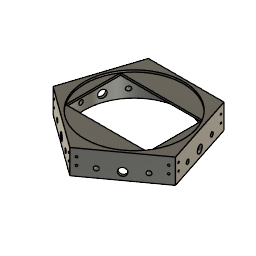
StarClock_InnerPart (Autodesk Fusion 360 design; units mm, degrees)
Autodesk Fusion 360 part; units mm, degrees
note: some values were not read from the file. Set by a fixed rule: which sketch regions a step uses.
sketch "Skizze1" plane through (0, 0, 0) normal (0, 0, 1) x (1, 0, 0)
  line L0 (0, -68.245) -> (64.9049, -21.0889)
  line L1 (64.9049, -21.0889) -> (40.1134, 55.2114)
  line L2 (40.1134, 55.2114) -> (-40.1134, 55.2114)
  line L3 (-40.1134, 55.2114) -> (-64.9049, -21.0889)
  line L4 (-64.9049, -21.0889) -> (0, -68.245)
  circle A0 centre (0, 0) radius 52.5
  line L5 (-43.5, 29) -> (43.5, 29)
  line L6 (43.5, 29) -> (43.5, -29)
  line L7 (43.5, -29) -> (-43.5, -29)
  line L8 (-43.5, -29) -> (-43.5, 29)
  line L9 (0, 0) -> (0, 29)
  line L10 (0, 29) -> (-43.5, 29)
  line L11 (0, -68.245) -> (0, -66.245)
  line L12 (0, -66.245) -> (63.0027, -20.4708)
  line L13 (63.0027, -20.4708) -> (38.9378, 53.5933)
  line L14 (38.9378, 53.5933) -> (-38.9378, 53.5933)
  line L15 (-38.9378, 53.5933) -> (-63.0027, -20.4708)
  line L16 (-63.0027, -20.4708) -> (0, -66.245)
  dimension "d1" = 68.245
  dimension "d2" = 105
  dimension "d3" = 87
  dimension "d4" = 58
  dimension "d5" = 29
  dimension "d6" = 43.5
  dimension "d7" = 2
  constraint coincident A0.centre L9.start
  constraint horizontal L5
  constraint vertical L6
  constraint horizontal L7
  constraint vertical L8
  constraint vertical L9
  constraint perpendicular L9 L10
  constraint vertical L11
  constraint coincident L11.end L12.start
  constraint coincident L9 A0.centre
  measures "d1" distance of L0.start A0.centre
  measures "d2" diameter of A0
  measures "d3" distance of L5.end L5.start
  measures "d4" distance of L7.end L5.start
  measures "d5" distance of A0.centre L9.end
  measures "d6" distance of L9.end L5.start
  measures "d7" distance of L0.start L11.end
extrude "Extrusion1" add sketch "Skizze1" along normal blind 12 and the other way blind 14 contours L0 L1 L2 L3 L4 | L12 L13 L14 L15 L16
extrude "Extrusion2" add sketch "Skizze1" along normal blind 2 from surface at 8 contours A0
sketch "Skizze2" plane through (32.4524, -44.6669, 0) normal (0.587785, -0.809017, 0) x (0.809017, 0.587785, 0)
  line L0 (40.1134, -14) -> (40.1134, 12)
  line L1 (40.1134, 12) -> (-40.1134, 12)
  line L2 (-40.1134, -14) -> (40.1134, -14)
  line L3 (0, -5) -> (-20, -5)
  circle A0 centre (-35, 4) radius 1
  line L4 (-35, -4) -> (-35, 4)
  line L5 (0, -12) -> (0, 12)
  circle A1 centre (-35, -4) radius 1
  line L6 (-35, 4) -> (-35, 12)
  line L7 (-35, -12) -> (-35, -4)
  circle A2 centre (-20, -5) radius 2.25
  line L8 (35, 4) -> (35, 12)
  circle A3 centre (35, -4) radius 1
  line L9 (35, -12) -> (35, -4)
  circle A4 centre (35, 4) radius 1
  line L10 (35, -4) -> (35, 4)
  line L11 (0, -5) -> (20, -5)
  circle A5 centre (20, -5) radius 2.25
  circle A6 centre (0, -6) radius 4
  point P0 (0, -5)
  dimension "d16" = 8
  dimension "d17" = 8
  dimension "d18" = 8
  dimension "d19" = 2
  dimension "d21" = 2
  dimension "d23" = 20
  dimension "d27" = 4.5
  constraint vertical L7
  constraint parallel L4 L7
  constraint parallel L4 L6
  constraint coincident L4.start A1.centre
  constraint coincident A0.centre L4.end
  constraint coincident P0 L3.start
  constraint perpendicular L3 L5
  constraint coincident L3.end A2.centre
  constraint symmetric L4.start L5 A3.centre
  constraint symmetric L6.end L5 L8.end
  constraint symmetric A0.centre L5 L8.start
  constraint symmetric L7.start L5 L9.start
  constraint symmetric L3.end L5 L11.end
  constraint symmetric P0 L5 L3.start
  constraint symmetric A0 L5 A4
  constraint symmetric L5 A1 A3
  constraint symmetric L5 A2 A5
  constraint coincident L5 A6.centre
  measures "d16" distance of L4.start L7.start
  measures "d17" distance of L4.start A0.centre
  measures "d18" distance of L6.end A0.centre
  measures "d19" diameter of A1
  measures "d21" diameter of A0
  measures "d23" distance of L3.end P0
  measures "d27" diameter of A2
extrude "Extrusion3" cut sketch "Skizze2" against normal blind 4 contours A0 L4 L6 | A0 L4 L6 | L4 A1 L7 | L4 A1 L7 | L8 A4 L10 | L8 A4 L10 | A3 L9 L10 | A3 L9 L10
extrude "Extrusion4" cut sketch "Skizze2" against normal blind 9 contours L3 L5 A6 | L5 L11 A6 | L3 L5 A6 | L5 L11 A6 | A2 | A5
sketch "Skizze3" plane through (32.4524, -44.6669, 0) normal (0.587785, -0.809017, 0) x (0.809017, 0.587785, 0)
sketch "Skizze4" plane through (52.5091, 17.0612, 0) normal (0.951057, 0.309017, 0) x (-0.309017, 0.951057, 0)
  line L0 (40.1134, -14) -> (40.1134, 12)
  line L1 (40.1134, 12) -> (-40.1134, 12)
  line L2 (-40.1134, 12) -> (-40.1134, -14)
  line L3 (-40.1134, -14) -> (40.1134, -14)
  line L4 (0, -5) -> (20, -5)
  line L5 (35, -4) -> (35, 4)
  line L6 (0, -5) -> (-20, -5)
  circle A0 centre (-20, -5) radius 2.25
  line L7 (35, 4) -> (35, 12)
  line L8 (40.1134, -12) -> (40.1134, 12)
  line L9 (-35, -4) -> (-35, 4)
  line L10 (-35, 4) -> (-35, 12)
  circle A1 centre (35, -4) radius 1
  circle A2 centre (20, -5) radius 2.25
  circle A3 centre (35, 4) radius 1
  line L11 (35, -12) -> (35, -4)
  line L12 (-35, -12) -> (-35, -4)
  circle A4 centre (-35, -4) radius 1
  line L13 (0, -12) -> (0, 12)
  circle A5 centre (-35, 4) radius 1
  circle A6 centre (0, -6) radius 4
  point P0 (0, -5)
  dimension "d34" = 8
  dimension "d35" = 8
  dimension "d36" = 8
  dimension "d37" = 2
  dimension "d38" = 2
  dimension "d39" = 20
  dimension "d40" = 4.5
  constraint vertical L12
  constraint parallel L9 L12
  constraint parallel L9 L10
  constraint coincident L9.start L12.end
  constraint coincident L9.end L10.start
  constraint coincident P0 L4.start
  constraint perpendicular L6 L13
  constraint coincident L6.end A0.centre
  constraint symmetric L9.start L5.start L13
  constraint symmetric L10.end L7.end L13
  constraint symmetric L9.end L5.end L13
  constraint symmetric L12.start L11.start L13
  constraint symmetric L6.end L4.end L13
  constraint symmetric P0 L4.start L13
  constraint symmetric A3 L13 A5
  constraint symmetric A1 A4 L13
  constraint symmetric A0 A2 L13
  constraint coincident A6.centre L13
  measures "d34" distance of L12.start L9.start
  measures "d35" distance of L9.end L9.start
  measures "d36" distance of L9.end L10.end
  measures "d37" diameter of A4
  measures "d38" diameter of A5
  measures "d39" distance of L6.end P0
  measures "d40" diameter of A0
sketch "Skizze5" plane through (0, 55.2114, 0) normal (0, 1, 0) x (-1, 0, 0)
  line L0 (40.1134, -14) -> (40.1134, 12)
  line L1 (40.1134, 12) -> (-40.1134, 12)
  line L2 (-40.1134, 12) -> (-40.1134, -14)
  line L3 (-40.1134, -14) -> (40.1134, -14)
  line L4 (0, -5) -> (20, -5)
  line L5 (35, -4) -> (35, 4)
  line L6 (0, -5) -> (-20, -5)
  circle A0 centre (-20, -5) radius 2.25
  line L7 (35, 4) -> (35, 12)
  line L8 (40.1134, -12) -> (40.1134, 12)
  line L9 (-35, -4) -> (-35, 4)
  line L10 (-35, 4) -> (-35, 12)
  circle A1 centre (35, -4) radius 1
  circle A2 centre (20, -5) radius 2.25
  circle A3 centre (35, 4) radius 1
  line L11 (35, -12) -> (35, -4)
  line L12 (-35, -12) -> (-35, -4)
  circle A4 centre (-35, -4) radius 1
  line L13 (0, -12) -> (0, 12)
  circle A5 centre (-35, 4) radius 1
  circle A6 centre (0, -6) radius 4
  point P0 (0, -5)
  dimension "d41" = 8
  dimension "d42" = 8
  dimension "d43" = 8
  dimension "d44" = 2
  dimension "d45" = 2
  dimension "d46" = 20
  dimension "d47" = 4.5
  constraint vertical L12
  constraint parallel L9 L12
  constraint parallel L9 L10
  constraint coincident L9.start L12.end
  constraint coincident L9.end L10.start
  constraint coincident P0 L4.start
  constraint perpendicular L6 L13
  constraint coincident L6.end A0.centre
  constraint symmetric L9.start L5.start L13
  constraint symmetric L10.end L7.end L13
  constraint symmetric L9.end L5.end L13
  constraint symmetric L12.start L11.start L13
  constraint symmetric L6.end L4.end L13
  constraint symmetric P0 L4.start L13
  constraint symmetric A3 L13 A5
  constraint symmetric A1 A4 L13
  constraint symmetric A0 A2 L13
  constraint coincident A6.centre L13
  measures "d41" distance of L12.start L9.start
  measures "d42" distance of L9.end L9.start
  measures "d43" distance of L9.end L10.end
  measures "d44" diameter of A4
  measures "d45" diameter of A5
  measures "d46" distance of L6.end P0
  measures "d47" diameter of A0
sketch "Skizze6" plane through (-52.5091, 17.0613, 0) normal (-0.951057, 0.309017, 0) x (-0.309017, -0.951057, 0)
  line L0 (40.1134, -14) -> (40.1134, 12)
  line L1 (40.1134, 12) -> (-40.1134, 12)
  line L2 (-40.1134, 12) -> (-40.1134, -14)
  line L3 (-40.1134, -14) -> (40.1134, -14)
  line L4 (0, -5) -> (20, -5)
  line L5 (35, -4) -> (35, 4)
  line L6 (0, -5) -> (-20, -5)
  circle A0 centre (-20, -5) radius 2.25
  line L7 (35, 4) -> (35, 12)
  line L8 (40.1134, -12) -> (40.1134, 12)
  line L9 (-35, -4) -> (-35, 4)
  line L10 (-35, 4) -> (-35, 12)
  circle A1 centre (35, -4) radius 1
  circle A2 centre (20, -5) radius 2.25
  circle A3 centre (35, 4) radius 1
  line L11 (35, -12) -> (35, -4)
  line L12 (-35, -12) -> (-35, -4)
  circle A4 centre (-35, -4) radius 1
  line L13 (0, -12) -> (0, 12)
  circle A5 centre (-35, 4) radius 1
  circle A6 centre (0, -6) radius 4
  point P0 (0, -5)
  dimension "d48" = 8
  dimension "d49" = 8
  dimension "d50" = 8
  dimension "d51" = 2
  dimension "d52" = 2
  dimension "d53" = 20
  dimension "d54" = 4.5
  constraint vertical L12
  constraint parallel L9 L12
  constraint parallel L9 L10
  constraint coincident L9.start L12.end
  constraint coincident L9.end L10.start
  constraint coincident P0 L4.start
  constraint perpendicular L6 L13
  constraint coincident L6.end A0.centre
  constraint symmetric L9.start L5.start L13
  constraint symmetric L10.end L7.end L13
  constraint symmetric L9.end L5.end L13
  constraint symmetric L12.start L11.start L13
  constraint symmetric L6.end L4.end L13
  constraint symmetric P0 L4.start L13
  constraint symmetric A3 L13 A5
  constraint symmetric A1 A4 L13
  constraint symmetric A0 A2 L13
  constraint coincident A6.centre L13
  measures "d48" distance of L12.start L9.start
  measures "d49" distance of L9.end L9.start
  measures "d50" distance of L9.end L10.end
  measures "d51" diameter of A4
  measures "d52" diameter of A5
  measures "d53" distance of L6.end P0
  measures "d54" diameter of A0
sketch "Skizze7" plane through (-32.4524, -44.6669, 0) normal (-0.587785, -0.809017, 0) x (0.809017, -0.587785, 0)
  line L0 (40.1134, -14) -> (40.1134, 12)
  line L1 (40.1134, 12) -> (-40.1134, 12)
  line L2 (-40.1134, 12) -> (-40.1134, -14)
  line L3 (-40.1134, -14) -> (40.1134, -14)
  line L4 (0, -5) -> (20, -5)
  line L5 (35, -4) -> (35, 4)
  line L6 (0, -5) -> (-20, -5)
  circle A0 centre (-20, -5) radius 2.25
  line L7 (35, 4) -> (35, 12)
  line L8 (40.1134, -12) -> (40.1134, 12)
  line L9 (-35, -4) -> (-35, 4)
  line L10 (-35, 4) -> (-35, 12)
  circle A1 centre (35, -4) radius 1
  circle A2 centre (20, -5) radius 2.25
  circle A3 centre (35, 4) radius 1
  line L11 (35, -12) -> (35, -4)
  line L12 (-35, -12) -> (-35, -4)
  circle A4 centre (-35, -4) radius 1
  line L13 (0, -12) -> (0, 12)
  circle A5 centre (-35, 4) radius 1
  circle A6 centre (0, -6) radius 4
  point P0 (0, -5)
  dimension "d55" = 8
  dimension "d56" = 8
  dimension "d57" = 8
  dimension "d58" = 2
  dimension "d59" = 2
  dimension "d60" = 20
  dimension "d61" = 4.5
  constraint vertical L12
  constraint parallel L9 L12
  constraint parallel L9 L10
  constraint coincident L9.start L12.end
  constraint coincident L9.end L10.start
  constraint coincident P0 L4.start
  constraint perpendicular L6 L13
  constraint coincident L6.end A0.centre
  constraint symmetric L9.start L5.start L13
  constraint symmetric L10.end L7.end L13
  constraint symmetric L9.end L5.end L13
  constraint symmetric L12.start L11.start L13
  constraint symmetric L6.end L4.end L13
  constraint symmetric P0 L4.start L13
  constraint symmetric A3 L13 A5
  constraint symmetric A1 A4 L13
  constraint symmetric A0 A2 L13
  constraint coincident A6.centre L13
  measures "d55" distance of L12.start L9.start
  measures "d56" distance of L9.end L9.start
  measures "d57" distance of L9.end L10.end
  measures "d58" diameter of A4
  measures "d59" diameter of A5
  measures "d60" distance of L6.end P0
  measures "d61" diameter of A0
extrude "Extrusion5" cut sketch "Skizze7" against normal blind 4 contours L5 A1 L11 | L5 A1 L11 | L5 L7 A3 | L5 L7 A3 | L9 L12 A4 | L9 L12 A4 | L9 L10 A5 | L9 L10 A5
extrude "Extrusion6" cut sketch "Skizze6" against normal blind 4 contours L5 A1 L11 | L5 A1 L11 | L5 L7 A3 | L5 L7 A3 | L9 L12 A4 | L9 L12 A4 | L9 L10 A5 | L9 L10 A5
extrude "Extrusion7" cut sketch "Skizze5" against normal blind 4 contours L5 A1 L11 | L5 A1 L11 | L5 L7 A3 | L5 L7 A3 | L9 L12 A4 | L9 L12 A4 | L9 L10 A5 | L9 L10 A5
extrude "Extrusion8" cut sketch "Skizze4" against normal blind 4 contours L5 A1 L11 | L5 A1 L11 | L5 L7 A3 | L5 L7 A3 | L9 L12 A4 | L9 L12 A4 | L9 L10 A5 | L9 L10 A5
extrude "Extrusion9" cut sketch "Skizze7" against normal blind 8 contours L4 L13 A6 | L6 L13 A6 | L4 L13 A6 | L6 L13 A6 | A0 | A2
extrude "Extrusion10" cut sketch "Skizze6" against normal blind 8 contours L4 L13 A6 | L6 L13 A6 | L4 L13 A6 | L6 L13 A6 | A0 | A2
extrude "Extrusion11" cut sketch "Skizze5" against normal blind 8 contours L4 L13 A6 | L6 L13 A6 | L4 L13 A6 | L6 L13 A6 | A0 | A2
extrude "Extrusion12" cut sketch "Skizze4" against normal blind 8 contours L4 L13 A6 | L6 L13 A6 | L4 L13 A6 | L6 L13 A6 | A0 | A2
sketch "Skizze8" plane through (0, 0, -14) normal (0, 0, -1) x (1, 0, 0)
  circle A0 centre (0, 0) radius 52.5
  line L0 (0, 68.245) -> (-64.9049, 21.0889)
  line L1 (-64.9049, 21.0889) -> (-40.1134, -55.2114)
  line L2 (-40.1134, -55.2114) -> (40.1134, -55.2114)
  line L3 (40.1134, -55.2114) -> (64.9049, 21.0889)
  line L4 (64.9049, 21.0889) -> (0, 68.245)
  line L5 (0, 0) -> (0, 68.245)
  line L6 (0, 0) -> (64.9049, 21.0889)
  line L7 (0, 0) -> (40.1134, -55.2114)
  line L8 (0, 0) -> (-40.1134, -55.2114)
  line L9 (0, 0) -> (-64.9049, 21.0889)
  line L10 (0, 0) -> (-57.0634, 18.541)
  line L11 (0, 0) -> (0, 60)
  line L12 (0, 0) -> (57.0634, 18.541)
  line L13 (0, 0) -> (35.2671, -48.541)
  line L14 (0, 0) -> (-35.2671, -48.541)
  circle A1 centre (-57.0634, 18.541) radius 1
  circle A2 centre (0, 60) radius 1
  circle A3 centre (57.0634, 18.541) radius 1
  circle A4 centre (35.2671, -48.541) radius 1
  circle A5 centre (-35.2671, -48.541) radius 1
  circle A6 centre (-57.0634, 18.541) radius 1.5
  circle A7 centre (0, 60) radius 1.5
  circle A8 centre (57.0634, 18.541) radius 1.5
  circle A9 centre (35.2671, -48.541) radius 1.5
  circle A10 centre (-35.2671, -48.541) radius 1.5
  dimension "d80" = 60
  dimension "d81" = 60
  dimension "d82" = 60
  dimension "d83" = 60
  dimension "d84" = 60
  dimension "d85" = 2
  dimension "d86" = 2
  dimension "d87" = 2
  dimension "d88" = 2
  dimension "d89" = 2
  dimension "d90" = 3
  dimension "d91" = 3
  dimension "d92" = 3
  dimension "d93" = 3
  dimension "d94" = 3
  constraint coincident A0.centre L5.start
  constraint coincident L0.start L4.end
  constraint coincident L3.end L4.start
  constraint coincident L2.end L3.start
  constraint coincident L1.end L2.start
  constraint coincident L0.end L1.start
  constraint parallel L9 L10
  constraint parallel L5 L11
  constraint parallel L6 L12
  constraint coincident L7 L13.end
  constraint coincident L8 L14.end
  constraint coincident L10.end A1.centre
  constraint coincident L11.end A2.centre
  constraint coincident L12.end A3.centre
  constraint coincident L13.end A4.centre
  constraint coincident L14.end A5.centre
  constraint concentric A1 A6
  constraint concentric A2 A7
  constraint concentric A3 A8
  constraint concentric A4 A9
  constraint concentric A5 A10
  measures "d80" distance of A0.centre L10.end
  measures "d81" distance of A0.centre L11.end
  measures "d82" distance of A0.centre L12.end
  measures "d83" distance of A0.centre L13.end
  measures "d84" distance of A0.centre L14.end
  measures "d85" diameter of A1
  measures "d86" diameter of A2
  measures "d87" diameter of A3
  measures "d88" diameter of A4
  measures "d89" diameter of A5
  measures "d90" diameter of A6
  measures "d91" diameter of A7
  measures "d92" diameter of A8
  measures "d93" diameter of A9
  measures "d94" diameter of A10
extrude "Extrusion13" cut sketch "Skizze8" against normal blind 8 contours L6 L12 A3 | L6 L12 A3 | L7 L13 A4 | L7 L13 A4 | L5 L11 A2 | L5 L11 A2 | L8 L14 A5 | L8 L14 A5 | L9 L10 A1 | L9 L10 A1
extrude "Extrusion14" cut sketch "Skizze8" against normal blind 2 contours L6 L12 A3 A8 | L6 L12 A3 A8 | L7 L13 A4 A9 | L7 L13 A4 A9 | L5 L11 A2 A7 | L5 L11 A2 A7 | L8 L14 A5 A10 | L8 L14 A5 A10 | L9 L10 A1 A6 | L9 L10 A1 A6
